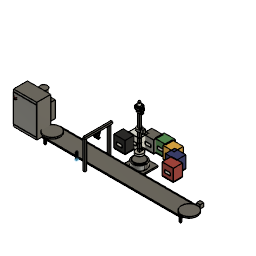
plastic_detector_model (Autodesk Fusion 360 design; units mm, degrees)
part number: 2026-06-23-12-15-38-462
part number: 2026-06-23-12-16-48-121
part number: 2026-06-23-12-16-48-324
part number: 2026-06-23-12-16-48-564
part number: 2026-06-23-12-16-48-693
part number: 2026-06-23-12-16-49-203
part number: 2026-06-23-12-16-49-677
part number: 2026-06-23-12-16-50-860
part number: 2026-06-23-12-16-51-924
part number: 2026-06-23-12-16-52-767
part number: 2026-06-23-12-24-08-550
part number: 2026-06-23-12-24-09-624
part number: 2026-06-23-12-24-10-773
part number: 2026-06-23-12-24-11-240
part number: 2026-06-23-12-24-12-927
part number: 2026-06-23-12-24-14-362
part number: 2026-06-23-12-24-17-480
part number: 2026-06-23-12-24-20-160
part number: 2026-06-23-12-24-22-024
part number: 2026-06-23-12-27-07-867
part number: 2026-06-23-12-27-09-721
part number: 2026-06-23-12-27-11-657
part number: 2026-06-23-12-27-12-541
part number: 2026-06-23-12-27-21-779
part number: 2026-06-23-12-27-31-682
part number: 2026-06-23-12-27-52-489
part number: 2026-06-23-12-28-09-652
part number: 2026-06-23-12-28-22-049
Autodesk Fusion 360 part; units mm, degrees
(part 1 of 3)
sketch "Sketch1" plane through (0, 0, 0) normal (0, 0, 1) x (1, 0, 0) in component "01_ConveyorBelt"
  line L0 (50, 0) -> (80, 0)
  line L1 (80, 0) -> (80, 30)
  line L2 (80, 30) -> (50, 30)
  line L3 (50, 30) -> (50, 0)
extrude "Extrude1" add sketch "Sketch1" along normal blind 100 makes body 1 in component "01_ConveyorBelt"
sketch "Sketch2" plane through (0, 0, 0) normal (0, 0, 1) x (1, 0, 0) in component "01_ConveyorBelt"
  line L0 (50, 370) -> (80, 370)
  line L1 (80, 370) -> (80, 400)
  line L2 (80, 400) -> (50, 400)
  line L3 (50, 400) -> (50, 370)
extrude "Extrude2" add sketch "Sketch2" along normal blind 100 separate body makes body 2 in component "01_ConveyorBelt"
sketch "Sketch3" plane through (0, 0, 0) normal (0, 0, 1) x (1, 0, 0) in component "01_ConveyorBelt"
  line L0 (2950, 0) -> (2980, 0)
  line L1 (2980, 0) -> (2980, 30)
  line L2 (2980, 30) -> (2950, 30)
  line L3 (2950, 30) -> (2950, 0)
extrude "Extrude3" add sketch "Sketch3" along normal blind 100 separate body makes body 3 in component "01_ConveyorBelt"
sketch "Sketch4" plane through (0, 0, 0) normal (0, 0, 1) x (1, 0, 0) in component "01_ConveyorBelt"
  line L0 (2950, 370) -> (2980, 370)
  line L1 (2980, 370) -> (2980, 400)
  line L2 (2980, 400) -> (2950, 400)
  line L3 (2950, 400) -> (2950, 370)
extrude "Extrude4" add sketch "Sketch4" along normal blind 100 separate body makes body 4 in component "01_ConveyorBelt"
sketch "Sketch5" plane through (0, 0, 0) normal (0, 0, 1) x (1, 0, 0) in component "01_ConveyorBelt"
  line L0 (0, 0, 100) -> (3000, 0, 100)
  line L1 (3000, 0, 100) -> (3000, 20, 100)
  line L2 (3000, 20, 100) -> (0, 20, 100)
  line L3 (0, 20, 100) -> (0, 0, 100)
extrude "Extrude5" add sketch "Sketch5" along normal blind 10 separate body contours L0 L1 L2 L3 in plane through (0, 0, 100) normal (0, 0, 1) makes body 5 in component "01_ConveyorBelt"
sketch "Sketch6" plane through (0, 0, 0) normal (0, 0, 1) x (1, 0, 0) in component "01_ConveyorBelt"
  line L0 (0, 380, 100) -> (3000, 380, 100)
  line L1 (3000, 380, 100) -> (3000, 400, 100)
  line L2 (3000, 400, 100) -> (0, 400, 100)
  line L3 (0, 400, 100) -> (0, 380, 100)
extrude "Extrude6" add sketch "Sketch6" along normal blind 10 separate body contours L0 L1 L2 L3 in plane through (0, 0, 100) normal (0, 0, 1) makes body 6 in component "01_ConveyorBelt"
sketch "Sketch7" plane through (0, 0, 0) normal (0, 0, 1) x (1, 0, 0) in component "01_ConveyorBelt"
  line L0 (0, 20, 100) -> (3000, 20, 100)
  line L1 (3000, 20, 100) -> (3000, 380, 100)
  line L2 (3000, 380, 100) -> (0, 380, 100)
  line L3 (0, 380, 100) -> (0, 20, 100)
extrude "Extrude7" add sketch "Sketch7" along normal blind 10 separate body contours L0 L1 L2 L3 in plane through (0, 0, 100) normal (0, 0, 1) makes body 7 in component "01_ConveyorBelt"
sketch "Sketch8" plane through (0, 0, 0) normal (0, 0, 1) x (1, 0, 0) in component "01_ConveyorBelt"
  circle A0 through (200, 200, 105) (-55, 347.2243, 105) (-55, 52.7757, 105)
extrude "Extrude8" add sketch "Sketch8" along normal blind 30 separate body contours A0 in plane through (0, 0, 105) normal (0, 0, 1) makes body 8 in component "01_ConveyorBelt"
sketch "Sketch9" plane through (0, 0, 0) normal (0, 0, 1) x (1, 0, 0) in component "01_ConveyorBelt"
  circle A0 through (3140, 200, 105) (2885, 347.2243, 105) (2885, 52.7757, 105)
extrude "Extrude9" add sketch "Sketch9" along normal blind 30 separate body contours A0 in plane through (0, 0, 105) normal (0, 0, 1) makes body 9 in component "01_ConveyorBelt"
sketch "Sketch10" plane through (0, 0, 0) normal (0, 0, 1) x (1, 0, 0) in component "01_ConveyorBelt"
  line L0 (2900, 420, 50) -> (2980, 420, 50)
  line L1 (2980, 420, 50) -> (2980, 500, 50)
  line L2 (2980, 500, 50) -> (2900, 500, 50)
  line L3 (2900, 500, 50) -> (2900, 420, 50)
extrude "Extrude10" add sketch "Sketch10" along normal blind 80 separate body contours L0 L1 L2 L3 in plane through (0, 0, 50) normal (0, 0, 1) makes body 10 in component "01_ConveyorBelt"
sketch "Sketch1 (2)" plane through (0, 0, 0) normal (0, 0, 1) x (1, 0, 0) in component "02_VisionStation"
  line L0 (970, -80) -> (1010, -80)
  line L1 (1010, -80) -> (1010, -40)
  line L2 (1010, -40) -> (970, -40)
  line L3 (970, -40) -> (970, -80)
extrude "Extrude1'" add sketch "Sketch1 (2)" along normal blind 600 separate body makes body 11 in component "02_VisionStation"
sketch "Sketch2 (2)" plane through (0, 0, 0) normal (0, 0, 1) x (1, 0, 0) in component "02_VisionStation"
  line L0 (970, 440) -> (1010, 440)
  line L1 (1010, 440) -> (1010, 480)
  line L2 (1010, 480) -> (970, 480)
  line L3 (970, 480) -> (970, 440)
extrude "Extrude2'" add sketch "Sketch2 (2)" along normal blind 600 separate body makes body 12 in component "02_VisionStation"
sketch "Sketch3 (2)" plane through (0, 0, 0) normal (0, 0, 1) x (1, 0, 0) in component "02_VisionStation"
  line L0 (970, -80, 600) -> (1010, -80, 600)
  line L1 (1010, -80, 600) -> (1010, 520, 600)
  line L2 (1010, 520, 600) -> (970, 520, 600)
  line L3 (970, 520, 600) -> (970, -80, 600)
extrude "Extrude3'" add sketch "Sketch3 (2)" along normal blind 40 separate body contours L0 L1 L2 L3 in plane through (0, 0, 600) normal (0, 0, 1) makes body 13 in component "02_VisionStation"
sketch "Sketch4 (2)" plane through (0, 0, 0) normal (0, 0, 1) x (1, 0, 0) in component "02_VisionStation"
  line L0 (960, 150, 580) -> (1020, 150, 580)
  line L1 (1020, 150, 580) -> (1020, 250, 580)
  line L2 (1020, 250, 580) -> (960, 250, 580)
  line L3 (960, 250, 580) -> (960, 150, 580)
extrude "Extrude4'" add sketch "Sketch4 (2)" along normal blind 20 separate body contours L0 L1 L2 L3 in plane through (0, 0, 580) normal (0, 0, 1) makes body 14 in component "02_VisionStation"
sketch "Sketch5 (2)" plane through (0, 0, 0) normal (0, 0, 1) x (1, 0, 0) in component "02_VisionStation"
  line L0 (965, 160, 540) -> (1015, 160, 540)
  line L1 (1015, 160, 540) -> (1015, 240, 540)
  line L2 (1015, 240, 540) -> (965, 240, 540)
  line L3 (965, 240, 540) -> (965, 160, 540)
extrude "Extrude5'" add sketch "Sketch5 (2)" along normal blind 40 separate body contours L0 L1 L2 L3 in plane through (0, 0, 540) normal (0, 0, 1) makes body 15 in component "02_VisionStation"
sketch "Sketch6 (2)" plane through (0, 0, 0) normal (0, 0, 1) x (1, 0, 0) in component "02_VisionStation"
  circle A0 through (1002, 200, 520) (984, 210.3923, 520) (984, 189.6077, 520)
extrude "Extrude6'" add sketch "Sketch6 (2)" along normal blind 20 separate body contours A0 in plane through (0, 0, 520) normal (0, 0, 1) makes body 16 in component "02_VisionStation"
sketch "Sketch7 (2)" plane through (0, 0, 0) normal (0, 0, 1) x (1, 0, 0) in component "02_VisionStation"
  line L0 (940, 180, 490) -> (1040, 180, 490)
  line L1 (1040, 180, 490) -> (1040, 220, 490)
  line L2 (1040, 220, 490) -> (940, 220, 490)
  line L3 (940, 220, 490) -> (940, 180, 490)
extrude "Extrude7'" add sketch "Sketch7 (2)" along normal blind 25 separate body contours L0 L1 L2 L3 in plane through (0, 0, 490) normal (0, 0, 1) makes body 17 in component "02_VisionStation"
sketch "Sketch8 (2)" plane through (0, 0, 0) normal (0, 0, 1) x (1, 0, 0) in component "02_VisionStation"
  circle A0 through (972, 195, 480) (961.5, 201.0622, 480) (961.5, 188.9378, 480)
extrude "Extrude8'" add sketch "Sketch8 (2)" along normal blind 10 separate body contours A0 in plane through (0, 0, 480) normal (0, 0, 1) makes body 18 in component "02_VisionStation"
sketch "Sketch9 (2)" plane through (0, 0, 0) normal (0, 0, 1) x (1, 0, 0) in component "02_VisionStation"
  circle A0 through (1022, 195, 480) (1011.5, 201.0622, 480) (1011.5, 188.9378, 480)
extrude "Extrude9'" add sketch "Sketch9 (2)" along normal blind 10 separate body contours A0 in plane through (0, 0, 480) normal (0, 0, 1) makes body 19 in component "02_VisionStation"
sketch "Sketch10 (2)" plane through (0, 0, 0) normal (0, 0, 1) x (1, 0, 0) in component "02_VisionStation"
  circle A0 through (1025, 200, 530) (972.5, 230.3109, 530) (972.5, 169.6891, 530)
extrude "Extrude10'" add sketch "Sketch10 (2)" along normal blind 5 separate body contours A0 in plane through (0, 0, 530) normal (0, 0, 1) makes body 20 in component "02_VisionStation"
sketch "Sketch1 (3)" plane through (0, 0, 0) normal (0, 0, 1) x (1, 0, 0) in component "03_RobotBase"
  line L0 (-200, -200) -> (200, -200)
  line L1 (200, -200) -> (200, 200)
  line L2 (200, 200) -> (-200, 200)
  line L3 (-200, 200) -> (-200, -200)
extrude "Extrude1''" add sketch "Sketch1 (3)" along normal blind 30 separate body makes body 21 in component "03_RobotBase"
sketch "Sketch2 (3)" plane through (0, 0, 0) normal (0, 0, 1) x (1, 0, 0) in component "03_RobotBase"
  circle A0 through (150, 0, 30) (-75, 129.9038, 30) (-75, -129.9038, 30)
extrude "Extrude2''" add sketch "Sketch2 (3)" along normal blind 100 separate body contours A0 in plane through (0, 0, 30) normal (0, 0, 1) makes body 22 in component "03_RobotBase"
sketch "Sketch3 (3)" plane through (0, 0, 0) normal (0, 0, 1) x (1, 0, 0) in component "03_RobotBase"
  circle A0 through (120, 0, 130) (-60, 103.923, 130) (-60, -103.923, 130)
extrude "Extrude3''" add sketch "Sketch3 (3)" along normal blind 20 separate body contours A0 in plane through (0, 0, 130) normal (0, 0, 1) makes body 23 in component "03_RobotBase"
sketch "Sketch4 (3)" plane through (0, 0, 0) normal (0, 0, 1) x (1, 0, 0) in component "03_RobotBase"
  line L0 (80, -40, 50) -> (136, -40, 50)
  line L1 (136, -40, 50) -> (136, 16, 50)
  line L2 (136, 16, 50) -> (80, 16, 50)
  line L3 (80, 16, 50) -> (80, -40, 50)
extrude "Extrude4''" add sketch "Sketch4 (3)" along normal blind 76 separate body contours L0 L1 L2 L3 in plane through (0, 0, 50) normal (0, 0, 1) makes body 24 in component "03_RobotBase"
sketch "Sketch1 (4)" plane through (0, 0, 0) normal (0, 0, 1) x (1, 0, 0) in component "04_RobotArm"
  circle A0 through (80, 0, 150) (-40, 69.282, 150) (-40, -69.282, 150)
extrude "Extrude1'''" add sketch "Sketch1 (4)" along normal blind 40 separate body contours A0 in plane through (0, 0, 150) normal (0, 0, 1) makes body 25 in component "04_RobotArm"
sketch "Sketch2 (4)" plane through (0, 0, 0) normal (0, 0, 1) x (1, 0, 0) in component "04_RobotArm"
  line L0 (-45, 50, 120) -> (11, 50, 120)
  line L1 (11, 50, 120) -> (11, 106, 120)
  line L2 (11, 106, 120) -> (-45, 106, 120)
  line L3 (-45, 106, 120) -> (-45, 50, 120)
extrude "Extrude2'''" add sketch "Sketch2 (4)" along normal blind 76 separate body contours L0 L1 L2 L3 in plane through (0, 0, 120) normal (0, 0, 1) makes body 26 in component "04_RobotArm"
sketch "Sketch3 (4)" plane through (0, 0, 0) normal (0, 0, 1) x (1, 0, 0) in component "04_RobotArm"
  line L0 (-20, -20, 190) -> (20, -20, 190)
  line L1 (20, -20, 190) -> (20, 20, 190)
  line L2 (20, 20, 190) -> (-20, 20, 190)
  line L3 (-20, 20, 190) -> (-20, -20, 190)
extrude "Extrude3'''" add sketch "Sketch3 (4)" along normal blind 400 separate body contours L0 L1 L2 L3 in plane through (0, 0, 190) normal (0, 0, 1) makes body 27 in component "04_RobotArm"
sketch "Sketch4 (4)" plane through (0, 0, 0) normal (0, 0, 1) x (1, 0, 0) in component "04_RobotArm"
  line L0 (-25, -25, 250) -> (25, -25, 250)
  line L1 (25, -25, 250) -> (25, 25, 250)
  line L2 (25, 25, 250) -> (-25, 25, 250)
  line L3 (-25, 25, 250) -> (-25, -25, 250)
extrude "Extrude4'''" add sketch "Sketch4 (4)" along normal blind 5 separate body contours L0 L1 L2 L3 in plane through (0, 0, 250) normal (0, 0, 1) makes body 28 in component "04_RobotArm"
sketch "Sketch5 (3)" plane through (0, 0, 0) normal (0, 0, 1) x (1, 0, 0) in component "04_RobotArm"
  line L0 (-25, -25, 350) -> (25, -25, 350)
  line L1 (25, -25, 350) -> (25, 25, 350)
  line L2 (25, 25, 350) -> (-25, 25, 350)
  line L3 (-25, 25, 350) -> (-25, -25, 350)
extrude "Extrude5''" add sketch "Sketch5 (3)" along normal blind 5 separate body contours L0 L1 L2 L3 in plane through (0, 0, 350) normal (0, 0, 1) makes body 29 in component "04_RobotArm"
sketch "Sketch6 (3)" plane through (0, 0, 0) normal (0, 0, 1) x (1, 0, 0) in component "04_RobotArm"
  line L0 (-25, -25, 450) -> (25, -25, 450)
  line L1 (25, -25, 450) -> (25, 25, 450)
  line L2 (25, 25, 450) -> (-25, 25, 450)
  line L3 (-25, 25, 450) -> (-25, -25, 450)
extrude "Extrude6''" add sketch "Sketch6 (3)" along normal blind 5 separate body contours L0 L1 L2 L3 in plane through (0, 0, 450) normal (0, 0, 1) makes body 30 in component "04_RobotArm"
sketch "Sketch7 (3)" plane through (0, 0, 0) normal (0, 0, 1) x (1, 0, 0) in component "04_RobotArm"
  circle A0 through (60, 0, 590) (-30, 51.9615, 590) (-30, -51.9615, 590)
extrude "Extrude7''" add sketch "Sketch7 (3)" along normal blind 40 separate body contours A0 in plane through (0, 0, 590) normal (0, 0, 1) makes body 31 in component "04_RobotArm"
sketch "Sketch8 (3)" plane through (0, 0, 0) normal (0, 0, 1) x (1, 0, 0) in component "04_RobotArm"
  line L0 (50, -30, 570) -> (106, -30, 570)
  line L1 (106, -30, 570) -> (106, 26, 570)
  line L2 (106, 26, 570) -> (50, 26, 570)
  line L3 (50, 26, 570) -> (50, -30, 570)
extrude "Extrude8''" add sketch "Sketch8 (3)" along normal blind 76 separate body contours L0 L1 L2 L3 in plane through (0, 0, 570) normal (0, 0, 1) makes body 32 in component "04_RobotArm"
sketch "Sketch9 (3)" plane through (0, 0, 0) normal (0, 0, 1) x (1, 0, 0) in component "04_RobotArm"
  line L0 (-20, -20, 630) -> (20, -20, 630)
  line L1 (20, -20, 630) -> (20, 20, 630)
  line L2 (20, 20, 630) -> (-20, 20, 630)
  line L3 (-20, 20, 630) -> (-20, -20, 630)
extrude "Extrude9''" add sketch "Sketch9 (3)" along normal blind 300 separate body contours L0 L1 L2 L3 in plane through (0, 0, 630) normal (0, 0, 1) makes body 33 in component "04_RobotArm"
sketch "Sketch10 (3)" plane through (0, 0, 0) normal (0, 0, 1) x (1, 0, 0) in component "04_RobotArm"
  circle A0 through (50, 0, 930) (-25, 43.3013, 930) (-25, -43.3013, 930)
extrude "Extrude10''" add sketch "Sketch10 (3)" along normal blind 30 separate body contours A0 in plane through (0, 0, 930) normal (0, 0, 1) makes body 34 in component "04_RobotArm"
sketch "Sketch11" plane through (0, 0, 0) normal (0, 0, 1) x (1, 0, 0) in component "04_RobotArm"
  line L0 (30, -20, 910) -> (70, -20, 910)
  line L1 (70, -20, 910) -> (70, 20, 910)
  line L2 (70, 20, 910) -> (30, 20, 910)
  line L3 (30, 20, 910) -> (30, -20, 910)
extrude "Extrude11" add sketch "Sketch11" along normal blind 50 separate body contours L0 L1 L2 L3 in plane through (0, 0, 910) normal (0, 0, 1) makes body 35 in component "04_RobotArm"
sketch "Sketch12" plane through (0, 0, 0) normal (0, 0, 1) x (1, 0, 0) in component "04_RobotArm"
  circle A0 through (-15, 30, 130) (-37.5, 42.9904, 130) (-37.5, 17.0096, 130)
extrude "Extrude12" add sketch "Sketch12" along normal blind 15 separate body contours A0 in plane through (0, 0, 130) normal (0, 0, 1) makes body 36 in component "04_RobotArm"
sketch "Sketch13" plane through (0, 0, 0) normal (0, 0, 1) x (1, 0, 0) in component "04_RobotArm"
  circle A0 through (-15, 30, 570) (-37.5, 42.9904, 570) (-37.5, 17.0096, 570)
extrude "Extrude13" add sketch "Sketch13" along normal blind 15 separate body contours A0 in plane through (0, 0, 570) normal (0, 0, 1) makes body 37 in component "04_RobotArm"
sketch "Sketch14" plane through (0, 0, 0) normal (0, 0, 1) x (1, 0, 0) in component "04_RobotArm"
  circle A0 through (-15, 30, 910) (-37.5, 42.9904, 910) (-37.5, 17.0096, 910)
extrude "Extrude14" add sketch "Sketch14" along normal blind 15 separate body contours A0 in plane through (0, 0, 910) normal (0, 0, 1) makes body 38 in component "04_RobotArm"
sketch "Sketch1 (5)" plane through (0, 0, 0) normal (0, 0, 1) x (1, 0, 0) in component "05_Gripper"
  line L0 (-50, -30) -> (50, -30)
  line L1 (50, -30) -> (50, 30)
  line L2 (50, 30) -> (-50, 30)
  line L3 (-50, 30) -> (-50, -30)
extrude "Extrude1''''" add sketch "Sketch1 (5)" along normal blind 60 separate body makes body 39 in component "05_Gripper"
sketch "Sketch2 (5)" plane through (0, 0, 0) normal (0, 0, 1) x (1, 0, 0) in component "05_Gripper"
  line L0 (-75, -30) -> (-50, -30)
  line L1 (-50, -30) -> (-50, 30)
  line L2 (-50, 30) -> (-75, 30)
  line L3 (-75, 30) -> (-75, -30)
extrude "Extrude2''''" add sketch "Sketch2 (5)" along normal blind 50 separate body makes body 40 in component "05_Gripper"
sketch "Sketch3 (5)" plane through (0, 0, 0) normal (0, 0, 1) x (1, 0, 0) in component "05_Gripper"
  line L0 (50, -30) -> (75, -30)
  line L1 (75, -30) -> (75, 30)
  line L2 (75, 30) -> (50, 30)
  line L3 (50, 30) -> (50, -30)
extrude "Extrude3''''" add sketch "Sketch3 (5)" along normal blind 50 separate body makes body 41 in component "05_Gripper"
sketch "Sketch4 (5)" plane through (0, 0, 0) normal (0, 0, 1) x (1, 0, 0) in component "05_Gripper"
  line L0 (-50, -25, 10) -> (50, -25, 10)
  line L1 (50, -25, 10) -> (50, -21, 10)
  line L2 (50, -21, 10) -> (-50, -21, 10)
  line L3 (-50, -21, 10) -> (-50, -25, 10)
extrude "Extrude4''''" add sketch "Sketch4 (5)" along normal blind 30 separate body contours L0 L1 L2 L3 in plane through (0, 0, 10) normal (0, 0, 1) makes body 42 in component "05_Gripper"
sketch "Sketch5 (4)" plane through (0, 0, 0) normal (0, 0, 1) x (1, 0, 0) in component "05_Gripper"
  line L0 (-50, 25, 10) -> (50, 25, 10)
  line L1 (50, 25, 10) -> (50, 29, 10)
  line L2 (50, 29, 10) -> (-50, 29, 10)
  line L3 (-50, 29, 10) -> (-50, 25, 10)
extrude "Extrude5'''" add sketch "Sketch5 (4)" along normal blind 30 separate body contours L0 L1 L2 L3 in plane through (0, 0, 10) normal (0, 0, 1) makes body 43 in component "05_Gripper"
sketch "Sketch6 (4)" plane through (0, 0, 0) normal (0, 0, 1) x (1, 0, 0) in component "05_Gripper"
  circle A0 through (25, 0, 60) (-12.5, 21.6506, 60) (-12.5, -21.6506, 60)
extrude "Extrude6'''" add sketch "Sketch6 (4)" along normal blind 80 separate body contours A0 in plane through (0, 0, 60) normal (0, 0, 1) makes body 44 in component "05_Gripper"
sketch "Sketch7 (4)" plane through (0, 0, 0) normal (0, 0, 1) x (1, 0, 0) in component "05_Gripper"
  circle A0 through (-16, 0, 140) (-22, 3.4641, 140) (-22, -3.4641, 140)
extrude "Extrude7'''" add sketch "Sketch7 (4)" along normal blind 30 separate body contours A0 in plane through (0, 0, 140) normal (0, 0, 1) makes body 45 in component "05_Gripper"
sketch "Sketch8 (4)" plane through (0, 0, 0) normal (0, 0, 1) x (1, 0, 0) in component "05_Gripper"
  circle A0 through (24, 0, 140) (18, 3.4641, 140) (18, -3.4641, 140)
extrude "Extrude8'''" add sketch "Sketch8 (4)" along normal blind 30 separate body contours A0 in plane through (0, 0, 140) normal (0, 0, 1) makes body 46 in component "05_Gripper"
sketch "Sketch9 (4)" plane through (0, 0, 0) normal (0, 0, 1) x (1, 0, 0) in component "05_Gripper"
  circle A0 through (30, 0, -20) (-15, 25.9808, -20) (-15, -25.9808, -20)
extrude "Extrude9'''" add sketch "Sketch9 (4)" along normal blind 20 separate body contours A0 in plane through (0, 0, -20) normal (0, 0, 1) makes body 47 in component "05_Gripper"
sketch "Sketch10 (4)" plane through (0, 0, 0) normal (0, 0, 1) x (1, 0, 0) in component "05_Gripper"
  line L0 (-10, -5, -5) -> (10, -5, -5)
  line L1 (10, -5, -5) -> (10, 5, -5)
  line L2 (10, 5, -5) -> (-10, 5, -5)
  line L3 (-10, 5, -5) -> (-10, -5, -5)
extrude "Extrude10'''" add sketch "Sketch10 (4)" along normal blind 3 separate body contours L0 L1 L2 L3 in plane through (0, 0, -5) normal (0, 0, 1) makes body 48 in component "05_Gripper"
sketch "Sketch11 (2)" plane through (0, 0, 0) normal (0, 0, 1) x (1, 0, 0) in component "05_Gripper"
  line L0 (-35, 35, 20) -> (35, 35, 20)
  line L1 (35, 35, 20) -> (35, 65, 20)
  line L2 (35, 65, 20) -> (-35, 65, 20)
  line L3 (-35, 65, 20) -> (-35, 35, 20)
extrude "Extrude11'" add sketch "Sketch11 (2)" along normal blind 40 separate body contours L0 L1 L2 L3 in plane through (0, 0, 20) normal (0, 0, 1) makes body 49 in component "05_Gripper"
sketch "Sketch1 (6)" plane through (0, 0, 0) normal (0, 0, 1) x (1, 0, 0) in component "06_SortingBins"
  line L0 (396.8309, 88.1111) -> (636.8309, 88.1111)
  line L1 (636.8309, 88.1111) -> (636.8309, 288.1111)
  line L2 (636.8309, 288.1111) -> (396.8309, 288.1111)
  line L3 (396.8309, 288.1111) -> (396.8309, 88.1111)
extrude "Extrude1'''''" add sketch "Sketch1 (6)" along normal blind 250 separate body makes body 50 in component "06_SortingBins"
sketch "Sketch2 (6)" plane through (0, 0, 0) normal (0, 0, 1) x (1, 0, 0) in component "06_SortingBins"
  line L0 (456.8309, 83.1111, 80) -> (576.8309, 83.1111, 80)
  line L1 (576.8309, 83.1111, 80) -> (576.8309, 86.1111, 80)
  line L2 (576.8309, 86.1111, 80) -> (456.8309, 86.1111, 80)
  line L3 (456.8309, 86.1111, 80) -> (456.8309, 83.1111, 80)
extrude "Extrude2'''''" add sketch "Sketch2 (6)" along normal blind 60 separate body contours L0 L1 L2 L3 in plane through (0, 0, 80) normal (0, 0, 1) makes body 51 in component "06_SortingBins"
sketch "Sketch3 (6)" plane through (0, 0, 0) normal (0, 0, 1) x (1, 0, 0) in component "06_SortingBins"
  line L0 (396.8309, 88.1111, -15) -> (636.8309, 88.1111, -15)
  line L1 (636.8309, 88.1111, -15) -> (636.8309, 288.1111, -15)
  line L2 (636.8309, 288.1111, -15) -> (396.8309, 288.1111, -15)
  line L3 (396.8309, 288.1111, -15) -> (396.8309, 88.1111, -15)
extrude "Extrude3'''''" add sketch "Sketch3 (6)" along normal blind 15 separate body contours L0 L1 L2 L3 in plane through (0, 0, -15) normal (0, 0, 1) makes body 52 in component "06_SortingBins"
sketch "Sketch4 (6)" plane through (0, 0, 0) normal (0, 0, 1) x (1, 0, 0) in component "06_SortingBins"
  line L0 (280.0555, 277.4329) -> (520.0555, 277.4329)
  line L1 (520.0555, 277.4329) -> (520.0555, 477.4329)
  line L2 (520.0555, 477.4329) -> (280.0555, 477.4329)
  line L3 (280.0555, 477.4329) -> (280.0555, 277.4329)
extrude "Extrude4'''''" add sketch "Sketch4 (6)" along normal blind 250 separate body makes body 53 in component "06_SortingBins"
sketch "Sketch5 (5)" plane through (0, 0, 0) normal (0, 0, 1) x (1, 0, 0) in component "06_SortingBins"
  line L0 (340.0555, 272.4329, 80) -> (460.0555, 272.4329, 80)
  line L1 (460.0555, 272.4329, 80) -> (460.0555, 275.4329, 80)
  line L2 (460.0555, 275.4329, 80) -> (340.0555, 275.4329, 80)
  line L3 (340.0555, 275.4329, 80) -> (340.0555, 272.4329, 80)
extrude "Extrude5''''" add sketch "Sketch5 (5)" along normal blind 60 separate body contours L0 L1 L2 L3 in plane through (0, 0, 80) normal (0, 0, 1) makes body 54 in component "06_SortingBins"
sketch "Sketch6 (5)" plane through (0, 0, 0) normal (0, 0, 1) x (1, 0, 0) in component "06_SortingBins"
  line L0 (280.0555, 277.4329, -15) -> (520.0555, 277.4329, -15)
  line L1 (520.0555, 277.4329, -15) -> (520.0555, 477.4329, -15)
  line L2 (520.0555, 477.4329, -15) -> (280.0555, 477.4329, -15)
  line L3 (280.0555, 477.4329, -15) -> (280.0555, 277.4329, -15)
extrude "Extrude6''''" add sketch "Sketch6 (5)" along normal blind 15 separate body contours L0 L1 L2 L3 in plane through (0, 0, -15) normal (0, 0, 1) makes body 55 in component "06_SortingBins"
sketch "Sketch7 (5)" plane through (0, 0, 0) normal (0, 0, 1) x (1, 0, 0) in component "06_SortingBins"
  line L0 (97.8439, 405.0189) -> (337.8439, 405.0189)
  line L1 (337.8439, 405.0189) -> (337.8439, 605.0189)
  line L2 (337.8439, 605.0189) -> (97.8439, 605.0189)
  line L3 (97.8439, 605.0189) -> (97.8439, 405.0189)
extrude "Extrude7''''" add sketch "Sketch7 (5)" along normal blind 250 separate body makes body 56 in component "06_SortingBins"
sketch "Sketch8 (5)" plane through (0, 0, 0) normal (0, 0, 1) x (1, 0, 0) in component "06_SortingBins"
  line L0 (157.8439, 400.0189, 80) -> (277.8439, 400.0189, 80)
  line L1 (277.8439, 400.0189, 80) -> (277.8439, 403.0189, 80)
  line L2 (277.8439, 403.0189, 80) -> (157.8439, 403.0189, 80)
  line L3 (157.8439, 403.0189, 80) -> (157.8439, 400.0189, 80)
extrude "Extrude8''''" add sketch "Sketch8 (5)" along normal blind 60 separate body contours L0 L1 L2 L3 in plane through (0, 0, 80) normal (0, 0, 1) makes body 57 in component "06_SortingBins"
sketch "Sketch9 (5)" plane through (0, 0, 0) normal (0, 0, 1) x (1, 0, 0) in component "06_SortingBins"
  line L0 (97.8439, 405.0189, -15) -> (337.8439, 405.0189, -15)
  line L1 (337.8439, 405.0189, -15) -> (337.8439, 605.0189, -15)
  line L2 (337.8439, 605.0189, -15) -> (97.8439, 605.0189, -15)
  line L3 (97.8439, 605.0189, -15) -> (97.8439, 405.0189, -15)
extrude "Extrude9''''" add sketch "Sketch9 (5)" along normal blind 15 separate body contours L0 L1 L2 L3 in plane through (0, 0, -15) normal (0, 0, 1) makes body 58 in component "06_SortingBins"
sketch "Sketch10 (5)" plane through (0, 0, 0) normal (0, 0, 1) x (1, 0, 0) in component "06_SortingBins"
  line L0 (-120, 450) -> (120, 450)
  line L1 (120, 450) -> (120, 650)
  line L2 (120, 650) -> (-120, 650)
  line L3 (-120, 650) -> (-120, 450)
extrude "Extrude10''''" add sketch "Sketch10 (5)" along normal blind 250 separate body makes body 59 in component "06_SortingBins"
sketch "Sketch11 (3)" plane through (0, 0, 0) normal (0, 0, 1) x (1, 0, 0) in component "06_SortingBins"
  line L0 (-60, 445, 80) -> (60, 445, 80)
  line L1 (60, 445, 80) -> (60, 448, 80)
  line L2 (60, 448, 80) -> (-60, 448, 80)
  line L3 (-60, 448, 80) -> (-60, 445, 80)
extrude "Extrude11''" add sketch "Sketch11 (3)" along normal blind 60 separate body contours L0 L1 L2 L3 in plane through (0, 0, 80) normal (0, 0, 1) makes body 60 in component "06_SortingBins"
sketch "Sketch12 (2)" plane through (0, 0, 0) normal (0, 0, 1) x (1, 0, 0) in component "06_SortingBins"
  line L0 (-120, 450, -15) -> (120, 450, -15)
  line L1 (120, 450, -15) -> (120, 650, -15)
  line L2 (120, 650, -15) -> (-120, 650, -15)
  line L3 (-120, 650, -15) -> (-120, 450, -15)
extrude "Extrude12'" add sketch "Sketch12 (2)" along normal blind 15 separate body contours L0 L1 L2 L3 in plane through (0, 0, -15) normal (0, 0, 1) makes body 61 in component "06_SortingBins"
sketch "Sketch13 (2)" plane through (0, 0, 0) normal (0, 0, 1) x (1, 0, 0) in component "06_SortingBins"
  line L0 (-337.8439, 405.0189) -> (-97.8439, 405.0189)
  line L1 (-97.8439, 405.0189) -> (-97.8439, 605.0189)
  line L2 (-97.8439, 605.0189) -> (-337.8439, 605.0189)
  line L3 (-337.8439, 605.0189) -> (-337.8439, 405.0189)
extrude "Extrude13'" add sketch "Sketch13 (2)" along normal blind 250 separate body makes body 62 in component "06_SortingBins"
sketch "Sketch14 (2)" plane through (0, 0, 0) normal (0, 0, 1) x (1, 0, 0) in component "06_SortingBins"
  line L0 (-277.8439, 400.0189, 80) -> (-157.8439, 400.0189, 80)
  line L1 (-157.8439, 400.0189, 80) -> (-157.8439, 403.0189, 80)
  line L2 (-157.8439, 403.0189, 80) -> (-277.8439, 403.0189, 80)
  line L3 (-277.8439, 403.0189, 80) -> (-277.8439, 400.0189, 80)
extrude "Extrude14'" add sketch "Sketch14 (2)" along normal blind 60 separate body contours L0 L1 L2 L3 in plane through (0, 0, 80) normal (0, 0, 1) makes body 63 in component "06_SortingBins"
sketch "Sketch15" plane through (0, 0, 0) normal (0, 0, 1) x (1, 0, 0) in component "06_SortingBins"
  line L0 (-337.8439, 405.0189, -15) -> (-97.8439, 405.0189, -15)
  line L1 (-97.8439, 405.0189, -15) -> (-97.8439, 605.0189, -15)
  line L2 (-97.8439, 605.0189, -15) -> (-337.8439, 605.0189, -15)
  line L3 (-337.8439, 605.0189, -15) -> (-337.8439, 405.0189, -15)
extrude "Extrude15" add sketch "Sketch15" along normal blind 15 separate body contours L0 L1 L2 L3 in plane through (0, 0, -15) normal (0, 0, 1) makes body 64 in component "06_SortingBins"
sketch "Sketch16" plane through (0, 0, 0) normal (0, 0, 1) x (1, 0, 0) in component "06_SortingBins"
  line L0 (-520.0555, 277.4329) -> (-280.0555, 277.4329)
  line L1 (-280.0555, 277.4329) -> (-280.0555, 477.4329)
  line L2 (-280.0555, 477.4329) -> (-520.0555, 477.4329)
  line L3 (-520.0555, 477.4329) -> (-520.0555, 277.4329)
extrude "Extrude16" add sketch "Sketch16" along normal blind 250 separate body makes body 65 in component "06_SortingBins"
sketch "Sketch17" plane through (0, 0, 0) normal (0, 0, 1) x (1, 0, 0) in component "06_SortingBins"
  line L0 (-460.0555, 272.4329, 80) -> (-340.0555, 272.4329, 80)
  line L1 (-340.0555, 272.4329, 80) -> (-340.0555, 275.4329, 80)
  line L2 (-340.0555, 275.4329, 80) -> (-460.0555, 275.4329, 80)
  line L3 (-460.0555, 275.4329, 80) -> (-460.0555, 272.4329, 80)
extrude "Extrude17" add sketch "Sketch17" along normal blind 60 separate body contours L0 L1 L2 L3 in plane through (0, 0, 80) normal (0, 0, 1) makes body 66 in component "06_SortingBins"
sketch "Sketch18" plane through (0, 0, 0) normal (0, 0, 1) x (1, 0, 0) in component "06_SortingBins"
  line L0 (-520.0555, 277.4329, -15) -> (-280.0555, 277.4329, -15)
  line L1 (-280.0555, 277.4329, -15) -> (-280.0555, 477.4329, -15)
  line L2 (-280.0555, 477.4329, -15) -> (-520.0555, 477.4329, -15)
  line L3 (-520.0555, 477.4329, -15) -> (-520.0555, 277.4329, -15)
extrude "Extrude18" add sketch "Sketch18" along normal blind 15 separate body contours L0 L1 L2 L3 in plane through (0, 0, -15) normal (0, 0, 1) makes body 67 in component "06_SortingBins"
sketch "Sketch19" plane through (0, 0, 0) normal (0, 0, 1) x (1, 0, 0) in component "06_SortingBins"
  line L0 (-636.8309, 88.1111) -> (-396.8309, 88.1111)
  line L1 (-396.8309, 88.1111) -> (-396.8309, 288.1111)
  line L2 (-396.8309, 288.1111) -> (-636.8309, 288.1111)
  line L3 (-636.8309, 288.1111) -> (-636.8309, 88.1111)
extrude "Extrude19" add sketch "Sketch19" along normal blind 250 separate body makes body 68 in component "06_SortingBins"
sketch "Sketch20" plane through (0, 0, 0) normal (0, 0, 1) x (1, 0, 0) in component "06_SortingBins"
  line L0 (-576.8309, 83.1111, 80) -> (-456.8309, 83.1111, 80)
  line L1 (-456.8309, 83.1111, 80) -> (-456.8309, 86.1111, 80)
  line L2 (-456.8309, 86.1111, 80) -> (-576.8309, 86.1111, 80)
  line L3 (-576.8309, 86.1111, 80) -> (-576.8309, 83.1111, 80)
extrude "Extrude20" add sketch "Sketch20" along normal blind 60 separate body contours L0 L1 L2 L3 in plane through (0, 0, 80) normal (0, 0, 1) makes body 69 in component "06_SortingBins"
sketch "Sketch21" plane through (0, 0, 0) normal (0, 0, 1) x (1, 0, 0) in component "06_SortingBins"
  line L0 (-636.8309, 88.1111, -15) -> (-396.8309, 88.1111, -15)
  line L1 (-396.8309, 88.1111, -15) -> (-396.8309, 288.1111, -15)
  line L2 (-396.8309, 288.1111, -15) -> (-636.8309, 288.1111, -15)
  line L3 (-636.8309, 288.1111, -15) -> (-636.8309, 88.1111, -15)
extrude "Extrude21" add sketch "Sketch21" along normal blind 15 separate body contours L0 L1 L2 L3 in plane through (0, 0, -15) normal (0, 0, 1) makes body 70 in component "06_SortingBins"
sketch "Sketch1 (7)" plane through (0, 0, 0) normal (0, 0, 1) x (1, 0, 0) in component "07_ComputeCabinet"
  line L0 (0, 0) -> (500, 0)
  line L1 (500, 0) -> (500, 300)
  line L2 (500, 300) -> (0, 300)
  line L3 (0, 300) -> (0, 0)
extrude "Extrude1''''''" add sketch "Sketch1 (7)" along normal blind 700 separate body makes body 71 in component "07_ComputeCabinet"
sketch "Sketch2 (7)" plane through (0, 0, 0) normal (0, 0, 1) x (1, 0, 0) in component "07_ComputeCabinet"
  line L0 (0, -5, 50) -> (500, -5, 50)
  line L1 (500, -5, 50) -> (500, 0, 50)
  line L2 (500, 0, 50) -> (0, 0, 50)
  line L3 (0, 0, 50) -> (0, -5, 50)
extrude "Extrude2''''''" add sketch "Sketch2 (7)" along normal blind 600 separate body contours L0 L1 L2 L3 in plane through (0, 0, 50) normal (0, 0, 1) makes body 72 in component "07_ComputeCabinet"
sketch "Sketch3 (7)" plane through (0, 0, 0) normal (0, 0, 1) x (1, 0, 0) in component "07_ComputeCabinet"
  line L0 (30, 50, 120) -> (470, 50, 120)
  line L1 (470, 50, 120) -> (470, 54, 120)
  line L2 (470, 54, 120) -> (30, 54, 120)
  line L3 (30, 54, 120) -> (30, 50, 120)
extrude "Extrude3''''''" add sketch "Sketch3 (7)" along normal blind 15 separate body contours L0 L1 L2 L3 in plane through (0, 0, 120) normal (0, 0, 1) makes body 73 in component "07_ComputeCabinet"
sketch "Sketch4 (7)" plane through (0, 0, 0) normal (0, 0, 1) x (1, 0, 0) in component "07_ComputeCabinet"
  line L0 (30, 50, 300) -> (470, 50, 300)
  line L1 (470, 50, 300) -> (470, 54, 300)
  line L2 (470, 54, 300) -> (30, 54, 300)
  line L3 (30, 54, 300) -> (30, 50, 300)
extrude "Extrude4''''''" add sketch "Sketch4 (7)" along normal blind 15 separate body contours L0 L1 L2 L3 in plane through (0, 0, 300) normal (0, 0, 1) makes body 74 in component "07_ComputeCabinet"
sketch "Sketch5 (6)" plane through (0, 0, 0) normal (0, 0, 1) x (1, 0, 0) in component "07_ComputeCabinet"
  line L0 (30, 50, 500) -> (470, 50, 500)
  line L1 (470, 50, 500) -> (470, 54, 500)
  line L2 (470, 54, 500) -> (30, 54, 500)
  line L3 (30, 54, 500) -> (30, 50, 500)
extrude "Extrude5'''''" add sketch "Sketch5 (6)" along normal blind 15 separate body contours L0 L1 L2 L3 in plane through (0, 0, 500) normal (0, 0, 1) makes body 75 in component "07_ComputeCabinet"
sketch "Sketch6 (6)" plane through (0, 0, 0) normal (0, 0, 1) x (1, 0, 0) in component "07_ComputeCabinet"
  line L0 (40, 60, 140) -> (140, 60, 140)
  line L1 (140, 60, 140) -> (140, 140, 140)
  line L2 (140, 140, 140) -> (40, 140, 140)
  line L3 (40, 140, 140) -> (40, 60, 140)
extrude "Extrude6'''''" add sketch "Sketch6 (6)" along normal blind 60 separate body contours L0 L1 L2 L3 in plane through (0, 0, 140) normal (0, 0, 1) makes body 76 in component "07_ComputeCabinet"
sketch "Sketch7 (6)" plane through (0, 0, 0) normal (0, 0, 1) x (1, 0, 0) in component "07_ComputeCabinet"
  circle A0 through (120, 100, 200) (75, 125.9808, 200) (75, 74.0192, 200)
extrude "Extrude7'''''" add sketch "Sketch7 (6)" along normal blind 10 separate body contours A0 in plane through (0, 0, 200) normal (0, 0, 1) makes body 77 in component "07_ComputeCabinet"
sketch "Sketch8 (6)" plane through (0, 0, 0) normal (0, 0, 1) x (1, 0, 0) in component "07_ComputeCabinet"
  line L0 (180, 60, 140) -> (240, 60, 140)
  line L1 (240, 60, 140) -> (240, 100, 140)
  line L2 (240, 100, 140) -> (180, 100, 140)
  line L3 (180, 100, 140) -> (180, 60, 140)
extrude "Extrude8'''''" add sketch "Sketch8 (6)" along normal blind 10 separate body contours L0 L1 L2 L3 in plane through (0, 0, 140) normal (0, 0, 1) makes body 78 in component "07_ComputeCabinet"
sketch "Sketch9 (6)" plane through (0, 0, 0) normal (0, 0, 1) x (1, 0, 0) in component "07_ComputeCabinet"
  line L0 (270, 60, 140) -> (350, 60, 140)
  line L1 (350, 60, 140) -> (350, 80, 140)
  line L2 (350, 80, 140) -> (270, 80, 140)
  line L3 (270, 80, 140) -> (270, 60, 140)
extrude "Extrude9'''''" add sketch "Sketch9 (6)" along normal blind 4 separate body contours L0 L1 L2 L3 in plane through (0, 0, 140) normal (0, 0, 1) makes body 79 in component "07_ComputeCabinet"
sketch "Sketch10 (6)" plane through (0, 0, 0) normal (0, 0, 1) x (1, 0, 0) in component "07_ComputeCabinet"
  line L0 (40, 60, 320) -> (220, 60, 320)
  line L1 (220, 60, 320) -> (220, 160, 320)
  line L2 (220, 160, 320) -> (40, 160, 320)
  line L3 (40, 160, 320) -> (40, 60, 320)
extrude "Extrude10'''''" add sketch "Sketch10 (6)" along normal blind 60 separate body contours L0 L1 L2 L3 in plane through (0, 0, 320) normal (0, 0, 1) makes body 80 in component "07_ComputeCabinet"
sketch "Sketch11 (4)" plane through (0, 0, 0) normal (0, 0, 1) x (1, 0, 0) in component "07_ComputeCabinet"
  line L0 (260, 60, 320) -> (440, 60, 320)
  line L1 (440, 60, 320) -> (440, 160, 320)
  line L2 (440, 160, 320) -> (260, 160, 320)
  line L3 (260, 160, 320) -> (260, 60, 320)
extrude "Extrude11'''" add sketch "Sketch11 (4)" along normal blind 60 separate body contours L0 L1 L2 L3 in plane through (0, 0, 320) normal (0, 0, 1) makes body 81 in component "07_ComputeCabinet"
sketch "Sketch12 (3)" plane through (0, 0, 0) normal (0, 0, 1) x (1, 0, 0) in component "07_ComputeCabinet"
  line L0 (40, 60, 520) -> (420, 60, 520)
  line L1 (420, 60, 520) -> (420, 200, 520)
  line L2 (420, 200, 520) -> (40, 200, 520)
  line L3 (40, 200, 520) -> (40, 60, 520)
extrude "Extrude12''" add sketch "Sketch12 (3)" along normal blind 100 separate body contours L0 L1 L2 L3 in plane through (0, 0, 520) normal (0, 0, 1) makes body 82 in component "07_ComputeCabinet"
sketch "Sketch13 (3)" plane through (0, 0, 0) normal (0, 0, 1) x (1, 0, 0) in component "07_ComputeCabinet"
  circle A0 through (80, -3, 550) (35, 22.9808, 550) (35, -28.9808, 550)
extrude "Extrude13''" add sketch "Sketch13 (3)" along normal blind 30 separate body contours A0 in plane through (0, 0, 550) normal (0, 0, 1) makes body 83 in component "07_ComputeCabinet"
sketch "Sketch14 (3)" plane through (0, 0, 0) normal (0, 0, 1) x (1, 0, 0) in component "07_ComputeCabinet"
  line L0 (360, 60, 140) -> (420, 60, 140)
  line L1 (420, 60, 140) -> (420, 100, 140)
  line L2 (420, 100, 140) -> (360, 100, 140)
  line L3 (360, 100, 140) -> (360, 60, 140)
extrude "Extrude14''" add sketch "Sketch14 (3)" along normal blind 40 separate body contours L0 L1 L2 L3 in plane through (0, 0, 140) normal (0, 0, 1) makes body 84 in component "07_ComputeCabinet"
sketch "Sketch15 (2)" plane through (0, 0, 0) normal (0, 0, 1) x (1, 0, 0) in component "07_ComputeCabinet"
  line L0 (180, 60, 220) -> (220, 60, 220)
  line L1 (220, 60, 220) -> (220, 85, 220)
  line L2 (220, 85, 220) -> (180, 85, 220)
  line L3 (180, 85, 220) -> (180, 60, 220)
extrude "Extrude15'" add sketch "Sketch15 (2)" along normal blind 3 separate body contours L0 L1 L2 L3 in plane through (0, 0, 220) normal (0, 0, 1) makes body 85 in component "07_ComputeCabinet"
sketch "Sketch1 (8)" plane through (0, 0, 0) normal (0, 0, 1) x (1, 0, 0) in component "08_PneumaticSystem"
  line L0 (0, 0) -> (300, 0)
  line L1 (300, 0) -> (300, 200)
  line L2 (300, 200) -> (0, 200)
  line L3 (0, 200) -> (0, 0)
extrude "Extrude1'''''''" add sketch "Sketch1 (8)" along normal blind 350 separate body makes body 86 in component "08_PneumaticSystem"
sketch "Sketch2 (8)" plane through (0, 0, 0) normal (0, 0, 1) x (1, 0, 0) in component "08_PneumaticSystem"
  circle A0 through (230, 100, 350) (110, 169.282, 350) (110, 30.718, 350)
extrude "Extrude2'''''''" add sketch "Sketch2 (8)" along normal blind 200 separate body contours A0 in plane through (0, 0, 350) normal (0, 0, 1) makes body 87 in component "08_PneumaticSystem"
sketch "Sketch3 (8)" plane through (0, 0, 0) normal (0, 0, 1) x (1, 0, 0) in component "08_PneumaticSystem"
  line L0 (0, 220, 150) -> (200, 220, 150)
  line L1 (200, 220, 150) -> (200, 300, 150)
  line L2 (200, 300, 150) -> (0, 300, 150)
  line L3 (0, 300, 150) -> (0, 220, 150)
extrude "Extrude3'''''''" add sketch "Sketch3 (8)" along normal blind 60 separate body contours L0 L1 L2 L3 in plane through (0, 0, 150) normal (0, 0, 1) makes body 88 in component "08_PneumaticSystem"
sketch "Sketch4 (8)" plane through (0, 0, 0) normal (0, 0, 1) x (1, 0, 0) in component "08_PneumaticSystem"
  line L0 (20, 220, 210) -> (60, 220, 210)
  line L1 (60, 220, 210) -> (60, 280, 210)
  line L2 (60, 280, 210) -> (20, 280, 210)
  line L3 (20, 280, 210) -> (20, 220, 210)
extrude "Extrude4'''''''" add sketch "Sketch4 (8)" along normal blind 40 separate body contours L0 L1 L2 L3 in plane through (0, 0, 210) normal (0, 0, 1) makes body 89 in component "08_PneumaticSystem"
sketch "Sketch5 (7)" plane through (0, 0, 0) normal (0, 0, 1) x (1, 0, 0) in component "08_PneumaticSystem"
  line L0 (80, 220, 210) -> (120, 220, 210)
  line L1 (120, 220, 210) -> (120, 280, 210)
  line L2 (120, 280, 210) -> (80, 280, 210)
  line L3 (80, 280, 210) -> (80, 220, 210)
extrude "Extrude5''''''" add sketch "Sketch5 (7)" along normal blind 40 separate body contours L0 L1 L2 L3 in plane through (0, 0, 210) normal (0, 0, 1) makes body 90 in component "08_PneumaticSystem"
sketch "Sketch6 (7)" plane through (0, 0, 0) normal (0, 0, 1) x (1, 0, 0) in component "08_PneumaticSystem"
  line L0 (140, 220, 210) -> (180, 220, 210)
  line L1 (180, 220, 210) -> (180, 280, 210)
  line L2 (180, 280, 210) -> (140, 280, 210)
  line L3 (140, 280, 210) -> (140, 220, 210)
extrude "Extrude6''''''" add sketch "Sketch6 (7)" along normal blind 40 separate body contours L0 L1 L2 L3 in plane through (0, 0, 210) normal (0, 0, 1) makes body 91 in component "08_PneumaticSystem"
sketch "Sketch7 (7)" plane through (0, 0, 0) normal (0, 0, 1) x (1, 0, 0) in component "08_PneumaticSystem"
  circle A0 through (195, 260, 150) (157.5, 281.6506, 150) (157.5, 238.3494, 150)
extrude "Extrude7''''''" add sketch "Sketch7 (7)" along normal blind 70 separate body contours A0 in plane through (0, 0, 150) normal (0, 0, 1) makes body 92 in component "08_PneumaticSystem"
sketch "Sketch8 (7)" plane through (0, 0, 0) normal (0, 0, 1) x (1, 0, 0) in component "08_PneumaticSystem"
  circle A0 through (50, 260, 150) (20, 277.3205, 150) (20, 242.6795, 150)
extrude "Extrude8''''''" add sketch "Sketch8 (7)" along normal blind 60 separate body contours A0 in plane through (0, 0, 150) normal (0, 0, 1) makes body 93 in component "08_PneumaticSystem"
sketch "Sketch9 (7)" plane through (0, 0, 0) normal (0, 0, 1) x (1, 0, 0) in component "08_PneumaticSystem"
  line L0 (200, 100, 200) -> (208, 100, 200)
  line L1 (208, 100, 200) -> (208, 250, 200)
  line L2 (208, 250, 200) -> (200, 250, 200)
  line L3 (200, 250, 200) -> (200, 100, 200)
extrude "Extrude9''''''" add sketch "Sketch9 (7)" along normal blind 8 separate body contours L0 L1 L2 L3 in plane through (0, 0, 200) normal (0, 0, 1) makes body 94 in component "08_PneumaticSystem"
sketch "Sketch10 (7)" plane through (0, 0, 0) normal (0, 0, 1) x (1, 0, 0) in component "08_PneumaticSystem"
  line L0 (230, 100, 200) -> (238, 100, 200)
  line L1 (238, 100, 200) -> (238, 250, 200)
  line L2 (238, 250, 200) -> (230, 250, 200)
  line L3 (230, 250, 200) -> (230, 100, 200)
extrude "Extrude10''''''" add sketch "Sketch10 (7)" along normal blind 8 separate body contours L0 L1 L2 L3 in plane through (0, 0, 200) normal (0, 0, 1) makes body 95 in component "08_PneumaticSystem"
sketch "Sketch1 (9)" plane through (0, 0, 0) normal (0, 0, 1) x (1, 0, 0) in component "09_TriggerSensor"
  line L0 (780, -50, 100) -> (800, -50, 100)
  line L1 (800, -50, 100) -> (800, -20, 100)
  line L2 (800, -20, 100) -> (780, -20, 100)
  line L3 (780, -20, 100) -> (780, -50, 100)
extrude "Extrude1''''''''" add sketch "Sketch1 (9)" along normal blind 150 separate body contours L0 L1 L2 L3 in plane through (0, 0, 100) normal (0, 0, 1) makes body 96 in component "09_TriggerSensor"
sketch "Sketch2 (9)" plane through (0, 0, 0) normal (0, 0, 1) x (1, 0, 0) in component "09_TriggerSensor"
  line L0 (780, -50, 200) -> (800, -50, 200)
  line L1 (800, -50, 200) -> (800, -10, 200)
  line L2 (800, -10, 200) -> (780, -10, 200)
  line L3 (780, -10, 200) -> (780, -50, 200)
extrude "Extrude2''''''''" add sketch "Sketch2 (9)" along normal blind 40 separate body contours L0 L1 L2 L3 in plane through (0, 0, 200) normal (0, 0, 1) makes body 97 in component "09_TriggerSensor"
sketch "Sketch1 (10)" plane through (0, 0, 0) normal (0, 0, 1) x (1, 0, 0) in component "01_ConveyorBelt (1)"
  line L0 (50, 0) -> (80, 0)
  line L1 (80, 0) -> (80, 30)
  line L2 (80, 30) -> (50, 30)
  line L3 (50, 30) -> (50, 0)
extrude "Extrude1'''''''''" add sketch "Sketch1 (10)" along normal blind 100 separate body makes body 98 in component "01_ConveyorBelt (1)"
sketch "Sketch2 (10)" plane through (0, 0, 0) normal (0, 0, 1) x (1, 0, 0) in component "01_ConveyorBelt (1)"
  line L0 (50, 370) -> (80, 370)
  line L1 (80, 370) -> (80, 400)
  line L2 (80, 400) -> (50, 400)
  line L3 (50, 400) -> (50, 370)
extrude "Extrude2'''''''''" add sketch "Sketch2 (10)" along normal blind 100 separate body makes body 99 in component "01_ConveyorBelt (1)"
sketch "Sketch3 (9)" plane through (0, 0, 0) normal (0, 0, 1) x (1, 0, 0) in component "01_ConveyorBelt (1)"
  line L0 (2950, 0) -> (2980, 0)
  line L1 (2980, 0) -> (2980, 30)
  line L2 (2980, 30) -> (2950, 30)
  line L3 (2950, 30) -> (2950, 0)
extrude "Extrude3''''''''" add sketch "Sketch3 (9)" along normal blind 100 separate body makes body 100 in component "01_ConveyorBelt (1)"
sketch "Sketch4 (9)" plane through (0, 0, 0) normal (0, 0, 1) x (1, 0, 0) in component "01_ConveyorBelt (1)"
  line L0 (2950, 370) -> (2980, 370)
  line L1 (2980, 370) -> (2980, 400)
  line L2 (2980, 400) -> (2950, 400)
  line L3 (2950, 400) -> (2950, 370)
extrude "Extrude4''''''''" add sketch "Sketch4 (9)" along normal blind 100 separate body makes body 101 in component "01_ConveyorBelt (1)"
sketch "Sketch5 (8)" plane through (0, 0, 0) normal (0, 0, 1) x (1, 0, 0) in component "01_ConveyorBelt (1)"
  line L0 (0, 0, 100) -> (3000, 0, 100)
  line L1 (3000, 0, 100) -> (3000, 20, 100)
  line L2 (3000, 20, 100) -> (0, 20, 100)
  line L3 (0, 20, 100) -> (0, 0, 100)
extrude "Extrude5'''''''" add sketch "Sketch5 (8)" along normal blind 10 separate body contours L0 L1 L2 L3 in plane through (0, 0, 100) normal (0, 0, 1) makes body 102 in component "01_ConveyorBelt (1)"
sketch "Sketch6 (8)" plane through (0, 0, 0) normal (0, 0, 1) x (1, 0, 0) in component "01_ConveyorBelt (1)"
  line L0 (0, 380, 100) -> (3000, 380, 100)
  line L1 (3000, 380, 100) -> (3000, 400, 100)
  line L2 (3000, 400, 100) -> (0, 400, 100)
  line L3 (0, 400, 100) -> (0, 380, 100)
extrude "Extrude6'''''''" add sketch "Sketch6 (8)" along normal blind 10 separate body contours L0 L1 L2 L3 in plane through (0, 0, 100) normal (0, 0, 1) makes body 103 in component "01_ConveyorBelt (1)"
sketch "Sketch7 (8)" plane through (0, 0, 0) normal (0, 0, 1) x (1, 0, 0) in component "01_ConveyorBelt (1)"
  line L0 (0, 20, 100) -> (3000, 20, 100)
  line L1 (3000, 20, 100) -> (3000, 380, 100)
  line L2 (3000, 380, 100) -> (0, 380, 100)
  line L3 (0, 380, 100) -> (0, 20, 100)
extrude "Extrude7'''''''" add sketch "Sketch7 (8)" along normal blind 10 separate body contours L0 L1 L2 L3 in plane through (0, 0, 100) normal (0, 0, 1) makes body 104 in component "01_ConveyorBelt (1)"
sketch "Sketch8 (8)" plane through (0, 0, 0) normal (0, 0, 1) x (1, 0, 0) in component "01_ConveyorBelt (1)"
  circle A0 through (200, 200, 105) (-55, 347.2243, 105) (-55, 52.7757, 105)
extrude "Extrude8'''''''" add sketch "Sketch8 (8)" along normal blind 30 separate body contours A0 in plane through (0, 0, 105) normal (0, 0, 1) makes body 105 in component "01_ConveyorBelt (1)"
sketch "Sketch9 (8)" plane through (0, 0, 0) normal (0, 0, 1) x (1, 0, 0) in component "01_ConveyorBelt (1)"
  circle A0 through (3140, 200, 105) (2885, 347.2243, 105) (2885, 52.7757, 105)
extrude "Extrude9'''''''" add sketch "Sketch9 (8)" along normal blind 30 separate body contours A0 in plane through (0, 0, 105) normal (0, 0, 1) makes body 106 in component "01_ConveyorBelt (1)"
sketch "Sketch10 (8)" plane through (0, 0, 0) normal (0, 0, 1) x (1, 0, 0) in component "01_ConveyorBelt (1)"
  line L0 (2900, 420, 50) -> (2980, 420, 50)
  line L1 (2980, 420, 50) -> (2980, 500, 50)
  line L2 (2980, 500, 50) -> (2900, 500, 50)
  line L3 (2900, 500, 50) -> (2900, 420, 50)
extrude "Extrude10'''''''" add sketch "Sketch10 (8)" along normal blind 80 separate body contours L0 L1 L2 L3 in plane through (0, 0, 50) normal (0, 0, 1) makes body 107 in component "01_ConveyorBelt (1)"
sketch "Sketch1 (11)" plane through (0, 0, 0) normal (0, 0, 1) x (1, 0, 0) in component "02_VisionStation (1)"
  line L0 (970, -80) -> (1010, -80)
  line L1 (1010, -80) -> (1010, -40)
  line L2 (1010, -40) -> (970, -40)
  line L3 (970, -40) -> (970, -80)
extrude "Extrude1''''''''''" add sketch "Sketch1 (11)" along normal blind 600 separate body makes body 108 in component "02_VisionStation (1)"
sketch "Sketch2 (11)" plane through (0, 0, 0) normal (0, 0, 1) x (1, 0, 0) in component "02_VisionStation (1)"
  line L0 (970, 440) -> (1010, 440)
  line L1 (1010, 440) -> (1010, 480)
  line L2 (1010, 480) -> (970, 480)
  line L3 (970, 480) -> (970, 440)
extrude "Extrude2''''''''''" add sketch "Sketch2 (11)" along normal blind 600 separate body makes body 109 in component "02_VisionStation (1)"
sketch "Sketch3 (10)" plane through (0, 0, 0) normal (0, 0, 1) x (1, 0, 0) in component "02_VisionStation (1)"
  line L0 (970, -80, 600) -> (1010, -80, 600)
  line L1 (1010, -80, 600) -> (1010, 520, 600)
  line L2 (1010, 520, 600) -> (970, 520, 600)
  line L3 (970, 520, 600) -> (970, -80, 600)
extrude "Extrude3'''''''''" add sketch "Sketch3 (10)" along normal blind 40 separate body contours L0 L1 L2 L3 in plane through (0, 0, 600) normal (0, 0, 1) makes body 110 in component "02_VisionStation (1)"
sketch "Sketch4 (10)" plane through (0, 0, 0) normal (0, 0, 1) x (1, 0, 0) in component "02_VisionStation (1)"
  line L0 (960, 150, 580) -> (1020, 150, 580)
  line L1 (1020, 150, 580) -> (1020, 250, 580)
  line L2 (1020, 250, 580) -> (960, 250, 580)
  line L3 (960, 250, 580) -> (960, 150, 580)